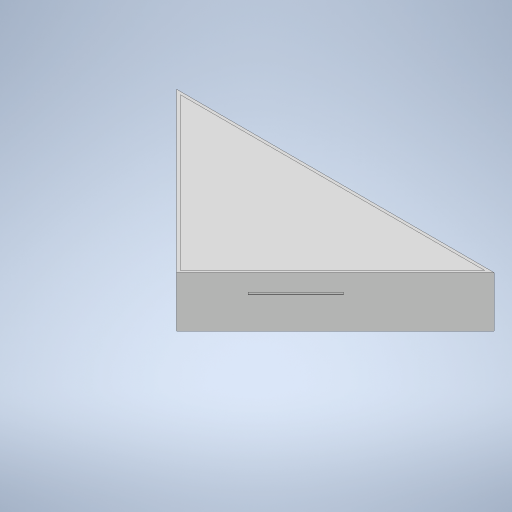
# Autodesk Inventor part: [Midterm]場地
Saved by Autodesk Inventor 2024 (Build 280153000, 153)
## iProperties
Created: 2024-04-14
Part Number: [Midterm]場地
Material: 一般
Document SubType Name: Modeling
Designer: USER
Density: 1 g/cm^3
Appearance: 預設
Author: USER
Autodesk Inventor part; units mm, degrees
ref_plane "YZ Plane" through (0, 0, 0) normal (1, 0, 0) x (0, 1, 0)
ref_plane "XZ Plane" through (0, 0, 0) normal (0, 1, 0) x (-1, 0, 0)
ref_plane "XY Plane" through (0, 0, 0) normal (0, 0, 1) x (1, 0, 0)
sketch "草圖1" plane through (0, 0, 0) normal (0, 1, 0) x (-1, 0, 0)
  line L0 (0, 0) -> (1200, 0)
  line L1 (1200, 0) -> (1200, -2100)
  line L2 (1200, -2100) -> (0, -2100)
  line L3 (0, -2100) -> (0, 0)
  line L4 (1200, -1900) -> (0, -1900)
  line L5 (1200, -1700) -> (0, -1700)
  line L6 (1200, -1500) -> (0, -1500)
  line L7 (1200, -1300) -> (0, -1300)
  line L8 (1200, 0) -> (600, 600)
  line L9 (0, 0) -> (600, 600)
  line L10 (1200, 0) -> (1700, -500)
  line L11 (0, 0) -> (-500, -500)
  line L12 (-500, -2100) -> (1700, -2100)
  line L13 (1700, -2100) -> (1700, -500)
  line L14 (-500, -500) -> (-500, -2100)
  line L15 (1700, -500) -> (3300, -2100)
  line L16 (3300, -2100) -> (1700, -2100)
  line L17 (-500, -2100) -> (-2100, -2100)
  line L18 (-2100, -2100) -> (-500, -500)
  line L19 (1735.3553, -464.6447) -> (3420.7107, -2150)
  line L20 (3420.7107, -2150) -> (1700, -2150)
  line L21 (-500, -2150) -> (1700, -2150)
  line L22 (-500, -2150) -> (-2220.7107, -2150)
  line L23 (-2220.7107, -2150) -> (-535.3553, -464.6447)
  line L24 (-35.3553, 35.3553) -> (-535.3553, -464.6447)
  line L25 (1235.3553, 35.3553) -> (600, 670.7107)
  line L26 (600, 670.7107) -> (-35.3553, 35.3553)
  line L27 (1235.3553, 35.3553) -> (1735.3553, -464.6447)
  point P0 (1700, 600)
  point P1 (-500, 600)
  point P2 (600, -2100)
  point P3 (600, -2100)
  point P4 (0, -2100)
  dimension "d0" = 2100
  dimension "d1" = 1200
  dimension "d2" = 200
  dimension "d3" = 200
  dimension "d4" = 200
  dimension "d5" = 200
  dimension "d6" = 45
  dimension "d7" = 45
  dimension "d8" = 500
  dimension "d9" = 45
  dimension "d19" = 50
  dimension "d20" = 50
  dimension "d21" = 50
  dimension "d22" = 50
  dimension "d23" = 50
  dimension "d24" = 50
  constraints: 56 end point, 9 point on line, 7 perpendicular, 6 parallel, 3 horizontal, 2 collinear, 2 horizontal alignment, 2 midpoint, 2 vertical alignment, 1 coincident, 3 other
  measures "d0" distance of L2.end L0.start
  measures "d1" distance of L0.start L0.end
  measures "d2" distance between parallel lines of L2 L4
  measures "d3" distance between parallel lines of L5 L4
  measures "d4" distance between parallel lines of L6 L5
  measures "d5" distance between parallel lines of L7 L6
  measures "d6" angle of L8 L0
  measures "d7" angle of L0 L9
  measures "d8" horizontal distance of L10.end L0.end
  measures "d9" angle of L1 L10
  measures "d19" distance between parallel lines of L15 L19
  measures "d20" distance between parallel lines of L12 L21
  measures "d21" distance between parallel lines of L17 L22
  measures "d22" distance between parallel lines of L11 L24
  measures "d23" distance between parallel lines of L8 L25
  measures "d24" distance between parallel lines of L10 L27
ref_plane "工作平面1" through (0, 0, 0) normal (0.7071068, 0, 0.7071068) x (0, 1, 0)
sketch "草圖2" plane through (0, 0, 0) normal (0.7071068, 0, 0.7071068) x (0, 1, 0)
  line L0 (0.1, 0) -> (600.1, 0)
  line L1 (600.1, 0) -> (600.1, -1200)
  line L2 (600.1, -1200) -> (0.1, -1200)
  line L3 (0.1, -1200) -> (0.1, 0)
  line L4 (560.1, 0) -> (560.1, -1200)
  point P0 (0, 0)
  point P1 (0.1, -600)
  dimension "d12" = 1200
  dimension "d13" = 600
  dimension "d14" = 40
  constraints: 10 end point, 2 parallel, 2 perpendicular, 2 point on line, 1 coincident, 1 horizontal, 1 midpoint
  measures "d12" distance of L0.end L1.end
  measures "d13" distance of L1.end L2.end
  measures "d14" distance between parallel lines of L4 L1
ref_plane "工作平面2" through (-1200, 0, 0) normal (0.7071068, 0, -0.7071068) x (-0.7071068, 0, -0.7071068)
sketch "草圖3" plane through (-1200, 0, 0) normal (0.7071068, 0, -0.7071068) x (-0.7071068, 0, -0.7071068)
  line L0 (1200, 0) -> (0, 0)
  line L1 (0, 0) -> (0, 600)
  line L2 (0, 600) -> (1200, 600)
  line L3 (1200, 600) -> (1200, 0)
  line L4 (1200, 560) -> (0, 560)
  point P0 (-848.5281, 0)
  point P1 (600, 0)
  dimension "d15" = 1200
  dimension "d16" = 600
  dimension "d17" = 40
  constraints: 10 end point, 2 parallel, 2 perpendicular, 2 point on line, 1 coincident, 1 horizontal, 1 midpoint
  measures "d15" distance of L1.end L2.end
  measures "d16" distance of L0.end L1.end
  measures "d17" distance between parallel lines of L2 L4
extrude "擠出2" add sketch "草圖1" along normal blind 900
sketch "草圖4" plane through (0, 900, 0) normal (0, 1, 0) x (1, 0, 0)
  line L0 (-600, -670.7107) -> (2220.7107, 2150) projected
  line L1 (2220.7107, 2150) -> (-3420.7107, 2150) projected
  line L2 (-600, -670.7107) -> (-3420.7107, 2150)
  line L3 (-3420.7107, 2150) -> (2220.7107, 2150)
  line L4 (2220.7107, 2150) -> (-600, -670.7107)
  line L5 (0, 0) -> (-600, -600) projected
  constraints: 6 end point, 1 collinear, 1 parallel
extrude "擠出3" add sketch "草圖4" along normal blind 0.1
extrude "擠出5" add sketch "草圖3" against normal blind 51 contours L4 L1 L2 L3
extrude "擠出6" add sketch "草圖2" along normal blind 51 contours L0 L1 L2 L4
